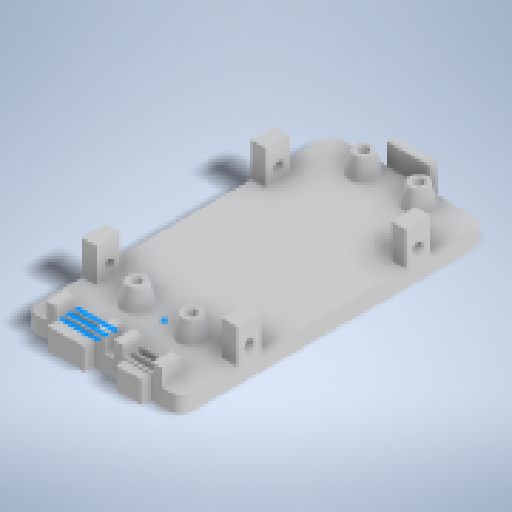
# Autodesk Inventor part: Base
Saved by Autodesk Inventor 2023 (Build 270158000, 158)
## iProperties
Created: 2022-06-08
Part Number: Base
Material: Generic
Document SubType Name: Modeling
Designer: siwat
Density: 1 g/cm^3
Appearance: Default
Author: siwat
Autodesk Inventor part; units mm, degrees
(part 1 of 3)
ref_plane "YZ Plane" through (0, 0, 0) normal (1, 0, 0) x (0, 1, 0)
ref_plane "XZ Plane" through (0, 0, 0) normal (0, 1, 0) x (-1, 0, 0)
ref_plane "XY Plane" through (0, 0, 0) normal (0, 0, 1) x (1, 0, 0)
sketch "Sketch1" plane through (0, 0, 0) normal (0, 1, 0) x (-1, 0, 0)
  line L0 (12.1706, 0.6153) -> (-9.8294, 0.6153)
  line L1 (-9.8294, 0.6153) -> (-9.8294, -51.3847)
  line L2 (-9.8294, -51.3847) -> (12.1706, -51.3847)
  line L3 (12.1706, -51.3847) -> (12.1706, 0.6153)
  line L4 (1.9706, -2.0847) -> (1.9706, 0.1153) projected
  arc A0 (1.7706, -2.2847) -> (1.9706, -2.0847) centre (1.7706, -2.0847) ccw projected
  line L5 (0.5706, -2.2847) -> (1.7706, -2.2847) projected
  arc A1 (0.3706, -2.0847) -> (0.5706, -2.2847) centre (0.5706, -2.0847) ccw projected
  line L6 (0.3706, 0.1153) -> (0.3706, -2.0847) projected
  line L7 (0.3706, 0.1153) -> (-0.5694, 0.1153) projected
  line L8 (-0.5694, -1.4847) -> (-0.5694, 0.1153) projected
  arc A2 (-2.1694, -1.4847) -> (-0.5694, -1.4847) centre (-1.3694, -1.4847) ccw projected
  line L9 (-2.1694, 0.1153) -> (-2.1694, -1.4847) projected
  line L10 (-2.1694, 0.1153) -> (-9.3294, 0.1153) projected
  line L11 (-9.3294, 0.1153) -> (-9.3294, -0.4547) projected
  line L12 (-9.3294, -0.4547) -> (-7.7294, -0.4547) projected
  arc A3 (-7.7294, -2.0547) -> (-7.7294, -0.4547) centre (-7.7294, -1.2547) ccw projected
  line L13 (-7.7294, -2.0547) -> (-9.3294, -2.0547) projected
  line L14 (-9.3294, -2.0547) -> (-9.3294, -2.9947) projected
  line L15 (-9.3294, -2.9947) -> (-7.7294, -2.9947) projected
  arc A4 (-7.7294, -4.5947) -> (-7.7294, -2.9947) centre (-7.7294, -3.7947) ccw projected
  line L16 (-7.7294, -4.5947) -> (-9.3294, -4.5947) projected
  line L17 (-9.3294, -4.5947) -> (-9.3294, -5.5347) projected
  line L18 (-9.3294, -5.5347) -> (-7.1294, -5.5347) projected
  arc A5 (-6.9294, -5.7347) -> (-7.1294, -5.5347) centre (-7.1294, -5.7347) ccw projected
  line L19 (-6.9294, -5.7347) -> (-6.9294, -6.9347) projected
  arc A6 (-7.1294, -7.1347) -> (-6.9294, -6.9347) centre (-7.1294, -6.9347) ccw projected
  line L20 (-7.1294, -7.1347) -> (-9.3294, -7.1347) projected
  line L21 (-9.3294, -7.1347) -> (-9.3294, -8.0747) projected
  line L22 (-9.3294, -8.0747) -> (-7.7294, -8.0747) projected
  arc A7 (-7.7294, -9.6747) -> (-7.7294, -8.0747) centre (-7.7294, -8.8747) ccw projected
  line L23 (-7.7294, -9.6747) -> (-9.3294, -9.6747) projected
  line L24 (-9.3294, -9.6747) -> (-9.3294, -10.6147) projected
  line L25 (-9.3294, -10.6147) -> (-7.7294, -10.6147) projected
  arc A8 (-7.7294, -12.2147) -> (-7.7294, -10.6147) centre (-7.7294, -11.4147) ccw projected
  line L26 (-7.7294, -12.2147) -> (-9.3294, -12.2147) projected
  line L27 (-9.3294, -12.2147) -> (-9.3294, -13.1547) projected
  line L28 (-9.3294, -13.1547) -> (-7.7294, -13.1547) projected
  arc A9 (-7.7294, -14.7547) -> (-7.7294, -13.1547) centre (-7.7294, -13.9547) ccw projected
  line L29 (-7.7294, -14.7547) -> (-9.3294, -14.7547) projected
  line L30 (-9.3294, -14.7547) -> (-9.3294, -15.6947) projected
  line L31 (-9.3294, -15.6947) -> (-7.7294, -15.6947) projected
  arc A10 (-7.7294, -17.2947) -> (-7.7294, -15.6947) centre (-7.7294, -16.4947) ccw projected
  line L32 (-7.7294, -17.2947) -> (-9.3294, -17.2947) projected
  line L33 (-9.3294, -17.2947) -> (-9.3294, -18.2347) projected
  line L34 (-9.3294, -18.2347) -> (-7.1294, -18.2347) projected
  arc A11 (-6.9294, -18.4347) -> (-7.1294, -18.2347) centre (-7.1294, -18.4347) ccw projected
  line L35 (-6.9294, -18.4347) -> (-6.9294, -19.6347) projected
  arc A12 (-7.1294, -19.8347) -> (-6.9294, -19.6347) centre (-7.1294, -19.6347) ccw projected
  line L36 (-7.1294, -19.8347) -> (-9.3294, -19.8347) projected
  line L37 (-9.3294, -19.8347) -> (-9.3294, -20.7747) projected
  line L38 (-9.3294, -20.7747) -> (-7.7294, -20.7747) projected
  arc A13 (-7.7294, -22.3747) -> (-7.7294, -20.7747) centre (-7.7294, -21.5747) ccw projected
  line L39 (-7.7294, -22.3747) -> (-9.3294, -22.3747) projected
  line L40 (-9.3294, -22.3747) -> (-9.3294, -23.3147) projected
  line L41 (-9.3294, -23.3147) -> (-7.7294, -23.3147) projected
  arc A14 (-7.7294, -24.9147) -> (-7.7294, -23.3147) centre (-7.7294, -24.1147) ccw projected
  line L42 (-7.7294, -24.9147) -> (-9.3294, -24.9147) projected
  line L43 (-9.3294, -24.9147) -> (-9.3294, -25.8547) projected
  line L44 (-9.3294, -25.8547) -> (-7.7294, -25.8547) projected
  arc A15 (-7.7294, -27.4547) -> (-7.7294, -25.8547) centre (-7.7294, -26.6547) ccw projected
  line L45 (-7.7294, -27.4547) -> (-9.3294, -27.4547) projected
  line L46 (-9.3294, -27.4547) -> (-9.3294, -28.3947) projected
  line L47 (-9.3294, -28.3947) -> (-7.7294, -28.3947) projected
  arc A16 (-7.7294, -29.9947) -> (-7.7294, -28.3947) centre (-7.7294, -29.1947) ccw projected
  line L48 (-7.7294, -29.9947) -> (-9.3294, -29.9947) projected
  line L49 (-9.3294, -29.9947) -> (-9.3294, -30.9347) projected
  line L50 (-9.3294, -30.9347) -> (-7.1294, -30.9347) projected
  arc A17 (-6.9294, -31.1347) -> (-7.1294, -30.9347) centre (-7.1294, -31.1347) ccw projected
  line L51 (-6.9294, -31.1347) -> (-6.9294, -32.3347) projected
  arc A18 (-7.1294, -32.5347) -> (-6.9294, -32.3347) centre (-7.1294, -32.3347) ccw projected
  line L52 (-7.1294, -32.5347) -> (-9.3294, -32.5347) projected
  line L53 (-9.3294, -32.5347) -> (-9.3294, -33.4747) projected
  line L54 (-9.3294, -33.4747) -> (-7.7294, -33.4747) projected
  arc A19 (-7.7294, -35.0747) -> (-7.7294, -33.4747) centre (-7.7294, -34.2747) ccw projected
  line L55 (-7.7294, -35.0747) -> (-9.3294, -35.0747) projected
  line L56 (-9.3294, -35.0747) -> (-9.3294, -36.0147) projected
  line L57 (-9.3294, -36.0147) -> (-7.7294, -36.0147) projected
  arc A20 (-7.7294, -37.6147) -> (-7.7294, -36.0147) centre (-7.7294, -36.8147) ccw projected
  line L58 (-7.7294, -37.6147) -> (-9.3294, -37.6147) projected
  line L59 (-9.3294, -37.6147) -> (-9.3294, -38.5547) projected
  line L60 (-9.3294, -38.5547) -> (-7.7294, -38.5547) projected
  arc A21 (-7.7294, -40.1547) -> (-7.7294, -38.5547) centre (-7.7294, -39.3547) ccw projected
  line L61 (-7.7294, -40.1547) -> (-9.3294, -40.1547) projected
  line L62 (-9.3294, -40.1547) -> (-9.3294, -41.0947) projected
  line L63 (-9.3294, -41.0947) -> (-7.7294, -41.0947) projected
  arc A22 (-7.7294, -42.6947) -> (-7.7294, -41.0947) centre (-7.7294, -41.8947) ccw projected
  line L64 (-7.7294, -42.6947) -> (-9.3294, -42.6947) projected
  line L65 (-9.3294, -42.6947) -> (-9.3294, -43.6347) projected
  line L66 (-9.3294, -43.6347) -> (-7.1294, -43.6347) projected
  arc A23 (-6.9294, -43.8347) -> (-7.1294, -43.6347) centre (-7.1294, -43.8347) ccw projected
  line L67 (-6.9294, -43.8347) -> (-6.9294, -45.0347) projected
  arc A24 (-7.1294, -45.2347) -> (-6.9294, -45.0347) centre (-7.1294, -45.0347) ccw projected
  line L68 (-7.1294, -45.2347) -> (-9.3294, -45.2347) projected
  line L69 (-9.3294, -45.2347) -> (-9.3294, -46.1747) projected
  line L70 (-9.3294, -46.1747) -> (-7.7294, -46.1747) projected
  arc A25 (-7.7294, -47.7747) -> (-7.7294, -46.1747) centre (-7.7294, -46.9747) ccw projected
  line L71 (-7.7294, -47.7747) -> (-9.3294, -47.7747) projected
  line L72 (-9.3294, -47.7747) -> (-9.3294, -48.7147) projected
  line L73 (-9.3294, -48.7147) -> (-7.7294, -48.7147) projected
  arc A26 (-7.7294, -50.3147) -> (-7.7294, -48.7147) centre (-7.7294, -49.5147) ccw projected
  line L74 (-7.7294, -50.3147) -> (-9.3294, -50.3147) projected
  line L75 (-9.3294, -50.3147) -> (-9.3294, -50.8847) projected
  line L76 (-9.3294, -50.8847) -> (11.6706, -50.8847) projected
  line L77 (11.6706, -50.8847) -> (11.6706, -50.3147) projected
  line L78 (10.0706, -50.3147) -> (11.6706, -50.3147) projected
  arc A27 (10.0706, -48.7147) -> (10.0706, -50.3147) centre (10.0706, -49.5147) ccw projected
  line L79 (11.6706, -48.7147) -> (10.0706, -48.7147) projected
  line L80 (11.6706, -48.7147) -> (11.6706, -47.7747) projected
  line L81 (10.0706, -47.7747) -> (11.6706, -47.7747) projected
  arc A28 (10.0706, -46.1747) -> (10.0706, -47.7747) centre (10.0706, -46.9747) ccw projected
  line L82 (11.6706, -46.1747) -> (10.0706, -46.1747) projected
  line L83 (11.6706, -46.1747) -> (11.6706, -45.2347) projected
  line L84 (9.4706, -45.2347) -> (11.6706, -45.2347) projected
  arc A29 (9.2706, -45.0347) -> (9.4706, -45.2347) centre (9.4706, -45.0347) ccw projected
  line L85 (9.2706, -43.8347) -> (9.2706, -45.0347) projected
  arc A30 (9.4706, -43.6347) -> (9.2706, -43.8347) centre (9.4706, -43.8347) ccw projected
  line L86 (11.6706, -43.6347) -> (9.4706, -43.6347) projected
  line L87 (11.6706, -43.6347) -> (11.6706, -42.6947) projected
  line L88 (10.0706, -42.6947) -> (11.6706, -42.6947) projected
  arc A31 (10.0706, -41.0947) -> (10.0706, -42.6947) centre (10.0706, -41.8947) ccw projected
  line L89 (11.6706, -41.0947) -> (10.0706, -41.0947) projected
  line L90 (11.6706, -41.0947) -> (11.6706, -40.1547) projected
  line L91 (10.0706, -40.1547) -> (11.6706, -40.1547) projected
  arc A32 (10.0706, -38.5547) -> (10.0706, -40.1547) centre (10.0706, -39.3547) ccw projected
  line L92 (11.6706, -38.5547) -> (10.0706, -38.5547) projected
  line L93 (11.6706, -38.5547) -> (11.6706, -37.6147) projected
  line L94 (10.0706, -37.6147) -> (11.6706, -37.6147) projected
  arc A33 (10.0706, -36.0147) -> (10.0706, -37.6147) centre (10.0706, -36.8147) ccw projected
  line L95 (11.6706, -36.0147) -> (10.0706, -36.0147) projected
  line L96 (11.6706, -36.0147) -> (11.6706, -35.0747) projected
  line L97 (10.0706, -35.0747) -> (11.6706, -35.0747) projected
  arc A34 (10.0706, -33.4747) -> (10.0706, -35.0747) centre (10.0706, -34.2747) ccw projected
  line L98 (11.6706, -33.4747) -> (10.0706, -33.4747) projected
  line L99 (11.6706, -33.4747) -> (11.6706, -32.5347) projected
  line L100 (9.4706, -32.5347) -> (11.6706, -32.5347) projected
  arc A35 (9.2706, -32.3347) -> (9.4706, -32.5347) centre (9.4706, -32.3347) ccw projected
  line L101 (9.2706, -31.1347) -> (9.2706, -32.3347) projected
  arc A36 (9.4706, -30.9347) -> (9.2706, -31.1347) centre (9.4706, -31.1347) ccw projected
  line L102 (11.6706, -30.9347) -> (9.4706, -30.9347) projected
  line L103 (11.6706, -30.9347) -> (11.6706, -29.9947) projected
  line L104 (10.0706, -29.9947) -> (11.6706, -29.9947) projected
  arc A37 (10.0706, -28.3947) -> (10.0706, -29.9947) centre (10.0706, -29.1947) ccw projected
  line L105 (11.6706, -28.3947) -> (10.0706, -28.3947) projected
  line L106 (11.6706, -28.3947) -> (11.6706, -27.4547) projected
  line L107 (10.0706, -27.4547) -> (11.6706, -27.4547) projected
  arc A38 (10.0706, -25.8547) -> (10.0706, -27.4547) centre (10.0706, -26.6547) ccw projected
  line L108 (11.6706, -25.8547) -> (10.0706, -25.8547) projected
  line L109 (11.6706, -25.8547) -> (11.6706, -24.9147) projected
  line L110 (10.0706, -24.9147) -> (11.6706, -24.9147) projected
  arc A39 (10.0706, -23.3147) -> (10.0706, -24.9147) centre (10.0706, -24.1147) ccw projected
  line L111 (11.6706, -23.3147) -> (10.0706, -23.3147) projected
  line L112 (11.6706, -23.3147) -> (11.6706, -22.3747) projected
  line L113 (10.0706, -22.3747) -> (11.6706, -22.3747) projected
  arc A40 (10.0706, -20.7747) -> (10.0706, -22.3747) centre (10.0706, -21.5747) ccw projected
  line L114 (11.6706, -20.7747) -> (10.0706, -20.7747) projected
  line L115 (11.6706, -20.7747) -> (11.6706, -19.8347) projected
  line L116 (9.4706, -19.8347) -> (11.6706, -19.8347) projected
  arc A41 (9.2706, -19.6347) -> (9.4706, -19.8347) centre (9.4706, -19.6347) ccw projected
  line L117 (9.2706, -18.4347) -> (9.2706, -19.6347) projected
  arc A42 (9.4706, -18.2347) -> (9.2706, -18.4347) centre (9.4706, -18.4347) ccw projected
  line L118 (11.6706, -18.2347) -> (9.4706, -18.2347) projected
  line L119 (11.6706, -18.2347) -> (11.6706, -17.2947) projected
  line L120 (10.0706, -17.2947) -> (11.6706, -17.2947) projected
  arc A43 (10.0706, -15.6947) -> (10.0706, -17.2947) centre (10.0706, -16.4947) ccw projected
  line L121 (11.6706, -15.6947) -> (10.0706, -15.6947) projected
  line L122 (11.6706, -15.6947) -> (11.6706, -14.7547) projected
  line L123 (10.0706, -14.7547) -> (11.6706, -14.7547) projected
  arc A44 (10.0706, -13.1547) -> (10.0706, -14.7547) centre (10.0706, -13.9547) ccw projected
  line L124 (11.6706, -13.1547) -> (10.0706, -13.1547) projected
  line L125 (11.6706, -13.1547) -> (11.6706, -12.2147) projected
  line L126 (10.0706, -12.2147) -> (11.6706, -12.2147) projected
  arc A45 (10.0706, -10.6147) -> (10.0706, -12.2147) centre (10.0706, -11.4147) ccw projected
  line L127 (11.6706, -10.6147) -> (10.0706, -10.6147) projected
  line L128 (11.6706, -10.6147) -> (11.6706, -9.6747) projected
  line L129 (10.0706, -9.6747) -> (11.6706, -9.6747) projected
  arc A46 (10.0706, -8.0747) -> (10.0706, -9.6747) centre (10.0706, -8.8747) ccw projected
  line L130 (11.6706, -8.0747) -> (10.0706, -8.0747) projected
  line L131 (11.6706, -8.0747) -> (11.6706, -7.1347) projected
  line L132 (9.4706, -7.1347) -> (11.6706, -7.1347) projected
  arc A47 (9.2706, -6.9347) -> (9.4706, -7.1347) centre (9.4706, -6.9347) ccw projected
  line L133 (9.2706, -5.7347) -> (9.2706, -6.9347) projected
  arc A48 (9.4706, -5.5347) -> (9.2706, -5.7347) centre (9.4706, -5.7347) ccw projected
  line L134 (11.6706, -5.5347) -> (9.4706, -5.5347) projected
  line L135 (11.6706, -5.5347) -> (11.6706, -4.5947) projected
  line L136 (10.0706, -4.5947) -> (11.6706, -4.5947) projected
  arc A49 (10.0706, -2.9947) -> (10.0706, -4.5947) centre (10.0706, -3.7947) ccw projected
  line L137 (11.6706, -2.9947) -> (10.0706, -2.9947) projected
  line L138 (11.6706, -2.9947) -> (11.6706, -2.0547) projected
  line L139 (10.0706, -2.0547) -> (11.6706, -2.0547) projected
  arc A50 (10.0706, -0.4547) -> (10.0706, -2.0547) centre (10.0706, -1.2547) ccw projected
  line L140 (11.6706, -0.4547) -> (10.0706, -0.4547) projected
  line L141 (11.6706, -0.4547) -> (11.6706, 0.1153) projected
  line L142 (11.6706, 0.1153) -> (4.5106, 0.1153) projected
  line L143 (4.5106, -1.4847) -> (4.5106, 0.1153) projected
  arc A51 (2.9106, -1.4847) -> (4.5106, -1.4847) centre (3.7106, -1.4847) ccw projected
  line L144 (2.9106, 0.1153) -> (2.9106, -1.4847) projected
  line L145 (2.9106, 0.1153) -> (1.9706, 0.1153) projected
  circle A52 centre (-4.5294, -48.8847) radius 1.9 projected
  circle A53 centre (6.8706, -48.8847) radius 1.9 projected
  circle A54 centre (-4.5294, -1.8847) radius 1.9 projected
  circle A55 centre (6.8706, -1.8847) radius 1.9 projected
  line L146 (15.1706, -52.3847) -> (-12.8294, -52.3847)
  line L147 (-14.8294, -50.3847) -> (-14.8294, 8.6153)
  line L148 (-12.8294, 10.6153) -> (15.1706, 10.6153)
  line L149 (17.1706, 8.6153) -> (17.1706, -50.3847)
  arc A56 (17.1706, 8.6153) -> (15.1706, 10.6153) centre (15.1706, 8.6153) ccw
  arc A57 (-12.8294, 10.6153) -> (-14.8294, 8.6153) centre (-12.8294, 8.6153) ccw
  arc A58 (-14.8294, -50.3847) -> (-12.8294, -52.3847) centre (-12.8294, -50.3847) ccw
  arc A59 (15.1706, -52.3847) -> (17.1706, -50.3847) centre (15.1706, -50.3847) ccw
  circle A60 centre (-4.5294, -1.8847) radius 0.75
  circle A61 centre (6.8706, -1.8847) radius 0.75
  circle A62 centre (-4.5294, -48.8847) radius 0.75
  circle A63 centre (6.8706, -48.8847) radius 0.75
  point P0 (11.6706, -2.5247)
  point P1 (-9.3294, -48.2447)
  point P2 (17.1706, -52.3847)
  point P3 (-14.8294, 10.6153)
  point P4 (-14.8294, -52.3847)
  point P5 (17.1706, 10.6153)
  dimension "d0" = 0.5
  dimension "d1" = 0.5
  dimension "d2" = 0.5
  dimension "d3" = 0.5
  dimension "d4" = 1
  dimension "d5" = 5
  dimension "d6" = 5
  dimension "d7" = 10
  dimension "d10" = 2
  dimension "d11" = 1.5
  dimension "d12" = 1.5
  dimension "d13" = 1.5
  dimension "d14" = 1.5
  constraints: 16 end point, 8 centre point, 8 point on circle, 8 point on line, 8 tangent, 4 coincident, 4 parallel, 3 equal radius, 2 horizontal, 2 midpoint, 2 perpendicular
  measures "d0" distance from line of L3 point (11.671, -2.525)
  measures "d1" distance between parallel lines of L0 L142
  measures "d2" distance between parallel lines of L2 L76
  measures "d3" distance from line of point (-9.329, -48.245) L1
  measures "d4" distance between parallel lines of L146 L2
  measures "d5" distance between parallel lines of L3 L149
  measures "d6" distance between parallel lines of L147 L1
  measures "d7" distance between parallel lines of L148 L0
  measures "d10" radius of A56
  measures "d11" diameter of A60
  measures "d12" diameter of A61
  measures "d13" diameter of A62
  measures "d14" diameter of A63
extrude "Extrusion1" add sketch "Sketch1" against normal blind 3.5 contours L3 L2 L1 L0 | L4 L145 L144 A51 L143 L142 L141 L140 A50 L139 L138 L137 A49 L136 L135 L134 A48 L133 A47 L132 L131 L130 A46 L129 L128 L127 A45 L126 L125 L124 A44 L123 L122 L121 A43 L120 L119 L118 A42 L117 A41 L116 L115 L114 A40 L113 L112 L111 A39 L110 L109 L108 A38 L107 L106 L105 A37 L104 L103 L102 A36 L101 A35 L100 L99 L98 A34 L97 L96 L95 A33 L94 L93 L92 A32 L91 L90 L89 A31 L88 L87 L86 A30 L85 A29 L84 L83 L82 A28 L81 L80 L79 A27 L78 L77 L76 L75 L74 A26 L73 L72 L71 A25 L70 L69 L68 A24 L67 A23 L66 L65 L64 A22 L63 L62 L61 A21 L60 L59 L58 A20 L57 L56 L55 A19 L54 L53 L52 A18 L51 A17 L50 L49 L48 A16 L47 L46 L45 A15 L44 L43 L42 A14 L41 L40 L39 A13 L38 L37 L36 A12 L35 A11 L34 L33 L32 A10 L31 L30 L29 A9 L28 L27 L26 A8 L25 L24 L23 A7 L22 L21 L20 A6 L19 A5 L18 L17 L16 A4 L15 L14 L13 A3 L12 L11 L10 L9 A2 L8 L7 L6 A1 L5 A0 | A52 | A53 | A54 | A55 | L146 A58 L147 A57 L148 A56 L149 A59 | A60 | A61 | A62 | A63
sketch "Sketch2" plane through (0, 0, 0) normal (0, 1, 0) x (1, 0, 0)
  line L0 (-1.9706, 2.0847) -> (-1.9706, -0.1153) projected
  arc A0 (-1.7706, 2.2847) -> (-1.9706, 2.0847) centre (-1.7706, 2.0847) ccw projected
  line L1 (-0.5706, 2.2847) -> (-1.7706, 2.2847) projected
  arc A1 (-0.3706, 2.0847) -> (-0.5706, 2.2847) centre (-0.5706, 2.0847) ccw projected
  line L2 (-0.3706, -0.1153) -> (-0.3706, 2.0847) projected
  line L3 (-0.3706, -0.1153) -> (0.5694, -0.1153) projected
  line L4 (0.5694, 1.4847) -> (0.5694, -0.1153) projected
  arc A2 (2.1694, 1.4847) -> (0.5694, 1.4847) centre (1.3694, 1.4847) ccw projected
  line L5 (2.1694, -0.1153) -> (2.1694, 1.4847) projected
  line L6 (2.1694, -0.1153) -> (9.3294, -0.1153) projected
  line L7 (9.3294, -0.1153) -> (9.3294, 0.4547) projected
  line L8 (9.3294, 0.4547) -> (7.7294, 0.4547) projected
  arc A3 (7.7294, 2.0547) -> (7.7294, 0.4547) centre (7.7294, 1.2547) ccw projected
  line L9 (7.7294, 2.0547) -> (9.3294, 2.0547) projected
  line L10 (9.3294, 2.0547) -> (9.3294, 2.9947) projected
  line L11 (9.3294, 2.9947) -> (7.7294, 2.9947) projected
  arc A4 (7.7294, 4.5947) -> (7.7294, 2.9947) centre (7.7294, 3.7947) ccw projected
  line L12 (7.7294, 4.5947) -> (9.3294, 4.5947) projected
  line L13 (9.3294, 4.5947) -> (9.3294, 5.5347) projected
  line L14 (9.3294, 5.5347) -> (7.1294, 5.5347) projected
  arc A5 (6.9294, 5.7347) -> (7.1294, 5.5347) centre (7.1294, 5.7347) ccw projected
  line L15 (6.9294, 5.7347) -> (6.9294, 6.9347) projected
  arc A6 (7.1294, 7.1347) -> (6.9294, 6.9347) centre (7.1294, 6.9347) ccw projected
  line L16 (7.1294, 7.1347) -> (9.3294, 7.1347) projected
  line L17 (9.3294, 7.1347) -> (9.3294, 8.0747) projected
  line L18 (9.3294, 8.0747) -> (7.7294, 8.0747) projected
  arc A7 (7.7294, 9.6747) -> (7.7294, 8.0747) centre (7.7294, 8.8747) ccw projected
  line L19 (7.7294, 9.6747) -> (9.3294, 9.6747) projected
  line L20 (9.3294, 9.6747) -> (9.3294, 10.6147) projected
  line L21 (9.3294, 10.6147) -> (7.7294, 10.6147) projected
  arc A8 (7.7294, 12.2147) -> (7.7294, 10.6147) centre (7.7294, 11.4147) ccw projected
  line L22 (7.7294, 12.2147) -> (9.3294, 12.2147) projected
  line L23 (9.3294, 12.2147) -> (9.3294, 13.1547) projected
  line L24 (9.3294, 13.1547) -> (7.7294, 13.1547) projected
  arc A9 (7.7294, 14.7547) -> (7.7294, 13.1547) centre (7.7294, 13.9547) ccw projected
  line L25 (7.7294, 14.7547) -> (9.3294, 14.7547) projected
  line L26 (9.3294, 14.7547) -> (9.3294, 15.6947) projected
  line L27 (9.3294, 15.6947) -> (7.7294, 15.6947) projected
  arc A10 (7.7294, 17.2947) -> (7.7294, 15.6947) centre (7.7294, 16.4947) ccw projected
  line L28 (7.7294, 17.2947) -> (9.3294, 17.2947) projected
  line L29 (9.3294, 17.2947) -> (9.3294, 18.2347) projected
  line L30 (9.3294, 18.2347) -> (7.1294, 18.2347) projected
  arc A11 (6.9294, 18.4347) -> (7.1294, 18.2347) centre (7.1294, 18.4347) ccw projected
  line L31 (6.9294, 18.4347) -> (6.9294, 19.6347) projected
  arc A12 (7.1294, 19.8347) -> (6.9294, 19.6347) centre (7.1294, 19.6347) ccw projected
  line L32 (7.1294, 19.8347) -> (9.3294, 19.8347) projected
  line L33 (9.3294, 19.8347) -> (9.3294, 20.7747) projected
  line L34 (9.3294, 20.7747) -> (7.7294, 20.7747) projected
  arc A13 (7.7294, 22.3747) -> (7.7294, 20.7747) centre (7.7294, 21.5747) ccw projected
  line L35 (7.7294, 22.3747) -> (9.3294, 22.3747) projected
  line L36 (9.3294, 22.3747) -> (9.3294, 23.3147) projected
  line L37 (9.3294, 23.3147) -> (7.7294, 23.3147) projected
  arc A14 (7.7294, 24.9147) -> (7.7294, 23.3147) centre (7.7294, 24.1147) ccw projected
  line L38 (7.7294, 24.9147) -> (9.3294, 24.9147) projected
  line L39 (9.3294, 24.9147) -> (9.3294, 25.8547) projected
  line L40 (9.3294, 25.8547) -> (7.7294, 25.8547) projected
  arc A15 (7.7294, 27.4547) -> (7.7294, 25.8547) centre (7.7294, 26.6547) ccw projected
  line L41 (7.7294, 27.4547) -> (9.3294, 27.4547) projected
  line L42 (9.3294, 27.4547) -> (9.3294, 28.3947) projected
  line L43 (9.3294, 28.3947) -> (7.7294, 28.3947) projected
  arc A16 (7.7294, 29.9947) -> (7.7294, 28.3947) centre (7.7294, 29.1947) ccw projected
  line L44 (7.7294, 29.9947) -> (9.3294, 29.9947) projected
  line L45 (9.3294, 29.9947) -> (9.3294, 30.9347) projected
  line L46 (9.3294, 30.9347) -> (7.1294, 30.9347) projected
  arc A17 (6.9294, 31.1347) -> (7.1294, 30.9347) centre (7.1294, 31.1347) ccw projected
  line L47 (6.9294, 31.1347) -> (6.9294, 32.3347) projected
  arc A18 (7.1294, 32.5347) -> (6.9294, 32.3347) centre (7.1294, 32.3347) ccw projected
  line L48 (7.1294, 32.5347) -> (9.3294, 32.5347) projected
  line L49 (9.3294, 32.5347) -> (9.3294, 33.4747) projected
  line L50 (9.3294, 33.4747) -> (7.7294, 33.4747) projected
  arc A19 (7.7294, 35.0747) -> (7.7294, 33.4747) centre (7.7294, 34.2747) ccw projected
  line L51 (7.7294, 35.0747) -> (9.3294, 35.0747) projected
  line L52 (9.3294, 35.0747) -> (9.3294, 36.0147) projected
  line L53 (9.3294, 36.0147) -> (7.7294, 36.0147) projected
  arc A20 (7.7294, 37.6147) -> (7.7294, 36.0147) centre (7.7294, 36.8147) ccw projected
  line L54 (7.7294, 37.6147) -> (9.3294, 37.6147) projected
  line L55 (9.3294, 37.6147) -> (9.3294, 38.5547) projected
  line L56 (9.3294, 38.5547) -> (7.7294, 38.5547) projected
  arc A21 (7.7294, 40.1547) -> (7.7294, 38.5547) centre (7.7294, 39.3547) ccw projected
  line L57 (7.7294, 40.1547) -> (9.3294, 40.1547) projected
  line L58 (9.3294, 40.1547) -> (9.3294, 41.0947) projected
  line L59 (9.3294, 41.0947) -> (7.7294, 41.0947) projected
  arc A22 (7.7294, 42.6947) -> (7.7294, 41.0947) centre (7.7294, 41.8947) ccw projected
  line L60 (7.7294, 42.6947) -> (9.3294, 42.6947) projected
  line L61 (9.3294, 42.6947) -> (9.3294, 43.6347) projected
  line L62 (9.3294, 43.6347) -> (7.1294, 43.6347) projected
  arc A23 (6.9294, 43.8347) -> (7.1294, 43.6347) centre (7.1294, 43.8347) ccw projected
  line L63 (6.9294, 43.8347) -> (6.9294, 45.0347) projected
  arc A24 (7.1294, 45.2347) -> (6.9294, 45.0347) centre (7.1294, 45.0347) ccw projected
  line L64 (7.1294, 45.2347) -> (9.3294, 45.2347) projected
  line L65 (9.3294, 45.2347) -> (9.3294, 46.1747) projected
  line L66 (9.3294, 46.1747) -> (7.7294, 46.1747) projected
  arc A25 (7.7294, 47.7747) -> (7.7294, 46.1747) centre (7.7294, 46.9747) ccw projected
  line L67 (7.7294, 47.7747) -> (9.3294, 47.7747) projected
  line L68 (9.3294, 47.7747) -> (9.3294, 48.7147) projected
  line L69 (9.3294, 48.7147) -> (7.7294, 48.7147) projected
  arc A26 (7.7294, 50.3147) -> (7.7294, 48.7147) centre (7.7294, 49.5147) ccw projected
  line L70 (7.7294, 50.3147) -> (9.3294, 50.3147) projected
  line L71 (9.3294, 50.3147) -> (9.3294, 50.8847) projected
  line L72 (9.3294, 50.8847) -> (-11.6706, 50.8847) projected
  line L73 (-11.6706, 50.8847) -> (-11.6706, 50.3147) projected
  line L74 (-10.0706, 50.3147) -> (-11.6706, 50.3147) projected
  arc A27 (-10.0706, 48.7147) -> (-10.0706, 50.3147) centre (-10.0706, 49.5147) ccw projected
  line L75 (-11.6706, 48.7147) -> (-10.0706, 48.7147) projected
  line L76 (-11.6706, 48.7147) -> (-11.6706, 47.7747) projected
  line L77 (-10.0706, 47.7747) -> (-11.6706, 47.7747) projected
  arc A28 (-10.0706, 46.1747) -> (-10.0706, 47.7747) centre (-10.0706, 46.9747) ccw projected
  line L78 (-11.6706, 46.1747) -> (-10.0706, 46.1747) projected
  line L79 (-11.6706, 46.1747) -> (-11.6706, 45.2347) projected
  line L80 (-9.4706, 45.2347) -> (-11.6706, 45.2347) projected
  arc A29 (-9.2706, 45.0347) -> (-9.4706, 45.2347) centre (-9.4706, 45.0347) ccw projected
  line L81 (-9.2706, 43.8347) -> (-9.2706, 45.0347) projected
  arc A30 (-9.4706, 43.6347) -> (-9.2706, 43.8347) centre (-9.4706, 43.8347) ccw projected
  line L82 (-11.6706, 43.6347) -> (-9.4706, 43.6347) projected
  line L83 (-11.6706, 43.6347) -> (-11.6706, 42.6947) projected
  line L84 (-10.0706, 42.6947) -> (-11.6706, 42.6947) projected
  arc A31 (-10.0706, 41.0947) -> (-10.0706, 42.6947) centre (-10.0706, 41.8947) ccw projected
  line L85 (-11.6706, 41.0947) -> (-10.0706, 41.0947) projected
  line L86 (-11.6706, 41.0947) -> (-11.6706, 40.1547) projected
  line L87 (-10.0706, 40.1547) -> (-11.6706, 40.1547) projected
  arc A32 (-10.0706, 38.5547) -> (-10.0706, 40.1547) centre (-10.0706, 39.3547) ccw projected
  line L88 (-11.6706, 38.5547) -> (-10.0706, 38.5547) projected
  line L89 (-11.6706, 38.5547) -> (-11.6706, 37.6147) projected
  line L90 (-10.0706, 37.6147) -> (-11.6706, 37.6147) projected
  arc A33 (-10.0706, 36.0147) -> (-10.0706, 37.6147) centre (-10.0706, 36.8147) ccw projected
  line L91 (-11.6706, 36.0147) -> (-10.0706, 36.0147) projected
  line L92 (-11.6706, 36.0147) -> (-11.6706, 35.0747) projected
  line L93 (-10.0706, 35.0747) -> (-11.6706, 35.0747) projected
  arc A34 (-10.0706, 33.4747) -> (-10.0706, 35.0747) centre (-10.0706, 34.2747) ccw projected
  line L94 (-11.6706, 33.4747) -> (-10.0706, 33.4747) projected
  line L95 (-11.6706, 33.4747) -> (-11.6706, 32.5347) projected
  line L96 (-9.4706, 32.5347) -> (-11.6706, 32.5347) projected
  arc A35 (-9.2706, 32.3347) -> (-9.4706, 32.5347) centre (-9.4706, 32.3347) ccw projected
  line L97 (-9.2706, 31.1347) -> (-9.2706, 32.3347) projected
  arc A36 (-9.4706, 30.9347) -> (-9.2706, 31.1347) centre (-9.4706, 31.1347) ccw projected
  line L98 (-11.6706, 30.9347) -> (-9.4706, 30.9347) projected
  line L99 (-11.6706, 30.9347) -> (-11.6706, 29.9947) projected
  line L100 (-10.0706, 29.9947) -> (-11.6706, 29.9947) projected
  arc A37 (-10.0706, 28.3947) -> (-10.0706, 29.9947) centre (-10.0706, 29.1947) ccw projected
  line L101 (-11.6706, 28.3947) -> (-10.0706, 28.3947) projected
  line L102 (-11.6706, 28.3947) -> (-11.6706, 27.4547) projected
  line L103 (-10.0706, 27.4547) -> (-11.6706, 27.4547) projected
  arc A38 (-10.0706, 25.8547) -> (-10.0706, 27.4547) centre (-10.0706, 26.6547) ccw projected
  line L104 (-11.6706, 25.8547) -> (-10.0706, 25.8547) projected
  line L105 (-11.6706, 25.8547) -> (-11.6706, 24.9147) projected
  line L106 (-10.0706, 24.9147) -> (-11.6706, 24.9147) projected
  arc A39 (-10.0706, 23.3147) -> (-10.0706, 24.9147) centre (-10.0706, 24.1147) ccw projected
  line L107 (-11.6706, 23.3147) -> (-10.0706, 23.3147) projected
  line L108 (-11.6706, 23.3147) -> (-11.6706, 22.3747) projected
  line L109 (-10.0706, 22.3747) -> (-11.6706, 22.3747) projected
  arc A40 (-10.0706, 20.7747) -> (-10.0706, 22.3747) centre (-10.0706, 21.5747) ccw projected
  line L110 (-11.6706, 20.7747) -> (-10.0706, 20.7747) projected
  line L111 (-11.6706, 20.7747) -> (-11.6706, 19.8347) projected
  line L112 (-9.4706, 19.8347) -> (-11.6706, 19.8347) projected
  arc A41 (-9.2706, 19.6347) -> (-9.4706, 19.8347) centre (-9.4706, 19.6347) ccw projected
  line L113 (-9.2706, 18.4347) -> (-9.2706, 19.6347) projected
  arc A42 (-9.4706, 18.2347) -> (-9.2706, 18.4347) centre (-9.4706, 18.4347) ccw projected
  line L114 (-11.6706, 18.2347) -> (-9.4706, 18.2347) projected
  line L115 (-11.6706, 18.2347) -> (-11.6706, 17.2947) projected
  line L116 (-10.0706, 17.2947) -> (-11.6706, 17.2947) projected
  arc A43 (-10.0706, 15.6947) -> (-10.0706, 17.2947) centre (-10.0706, 16.4947) ccw projected
  line L117 (-11.6706, 15.6947) -> (-10.0706, 15.6947) projected
  line L118 (-11.6706, 15.6947) -> (-11.6706, 14.7547) projected
  line L119 (-10.0706, 14.7547) -> (-11.6706, 14.7547) projected
  arc A44 (-10.0706, 13.1547) -> (-10.0706, 14.7547) centre (-10.0706, 13.9547) ccw projected
  line L120 (-11.6706, 13.1547) -> (-10.0706, 13.1547) projected
  line L121 (-11.6706, 13.1547) -> (-11.6706, 12.2147) projected
  line L122 (-10.0706, 12.2147) -> (-11.6706, 12.2147) projected
  arc A45 (-10.0706, 10.6147) -> (-10.0706, 12.2147) centre (-10.0706, 11.4147) ccw projected
  line L123 (-11.6706, 10.6147) -> (-10.0706, 10.6147) projected
  line L124 (-11.6706, 10.6147) -> (-11.6706, 9.6747) projected
  line L125 (-10.0706, 9.6747) -> (-11.6706, 9.6747) projected
  arc A46 (-10.0706, 8.0747) -> (-10.0706, 9.6747) centre (-10.0706, 8.8747) ccw projected
  line L126 (-11.6706, 8.0747) -> (-10.0706, 8.0747) projected
  line L127 (-11.6706, 8.0747) -> (-11.6706, 7.1347) projected
  line L128 (-9.4706, 7.1347) -> (-11.6706, 7.1347) projected
  arc A47 (-9.2706, 6.9347) -> (-9.4706, 7.1347) centre (-9.4706, 6.9347) ccw projected
  line L129 (-9.2706, 5.7347) -> (-9.2706, 6.9347) projected
  arc A48 (-9.4706, 5.5347) -> (-9.2706, 5.7347) centre (-9.4706, 5.7347) ccw projected
  line L130 (-11.6706, 5.5347) -> (-9.4706, 5.5347) projected
  line L131 (-11.6706, 5.5347) -> (-11.6706, 4.5947) projected
  line L132 (-10.0706, 4.5947) -> (-11.6706, 4.5947) projected
  arc A49 (-10.0706, 2.9947) -> (-10.0706, 4.5947) centre (-10.0706, 3.7947) ccw projected
  line L133 (-11.6706, 2.9947) -> (-10.0706, 2.9947) projected
  line L134 (-11.6706, 2.9947) -> (-11.6706, 2.0547) projected
  line L135 (-10.0706, 2.0547) -> (-11.6706, 2.0547) projected
  arc A50 (-10.0706, 0.4547) -> (-10.0706, 2.0547) centre (-10.0706, 1.2547) ccw projected
  line L136 (-11.6706, 0.4547) -> (-10.0706, 0.4547) projected
  line L137 (-11.6706, 0.4547) -> (-11.6706, -0.1153) projected
  line L138 (-11.6706, -0.1153) -> (-4.5106, -0.1153) projected
  line L139 (-4.5106, 1.4847) -> (-4.5106, -0.1153) projected
  arc A51 (-2.9106, 1.4847) -> (-4.5106, 1.4847) centre (-3.7106, 1.4847) ccw projected
  line L140 (-2.9106, -0.1153) -> (-2.9106, 1.4847) projected
  line L141 (-2.9106, -0.1153) -> (-1.9706, -0.1153) projected
  circle A52 centre (4.5294, 48.8847) radius 1.9 projected
  circle A53 centre (-6.8706, 48.8847) radius 1.9 projected
  circle A54 centre (4.5294, 1.8847) radius 1.9 projected
  circle A55 centre (-6.8706, 1.8847) radius 1.9 projected
  circle A56 centre (4.5294, 1.8847) radius 1.9
  circle A57 centre (-6.8706, 1.8847) radius 2
  circle A58 centre (-6.8706, 48.8847) radius 1.9
  circle A59 centre (4.5294, 48.8847) radius 1.9
  circle A60 centre (4.5294, 48.8847) radius 1
  circle A61 centre (-6.8706, 48.8847) radius 1
  circle A62 centre (4.5294, 1.8847) radius 1
  circle A63 centre (-6.8706, 1.8847) radius 1
  point P0 (0, 0)
  dimension "d15" = 2
  dimension "d16" = 2
  dimension "d17" = 2
  dimension "d18" = 2
  constraints: 8 centre point, 8 coincident, 3 concentric, 1 tangent
  measures "d15" diameter of A60
  measures "d16" diameter of A61
  measures "d17" diameter of A62
  measures "d18" diameter of A63
extrude "Extrusion2" add sketch "Sketch2" along normal blind 4 contours A52 | A53 | A54 | A55
chamfer "Chamfer1" distance 1 distance2 4 4 edges at (2.6294, 0, -48.8847) (-8.7706, 0, -48.8847) (-8.7706, 0, -1.8847) (2.6294, 0, -1.8847) measured on face at (2.1294, 0, -1.8847) measured on face at (-9.2706, 0, -1.8847) measured on face at (2.1294, 0, -48.8847) measured on face at (-9.2706, 0, -48.8847)
sketch "Sketch3" plane through (0, 0, 0) normal (0, 1, 0) x (1, 0, 0)
  line L0 (14.8294, 50.3847) -> (14.8294, -8.6153) projected
  line L1 (14.8294, 40.8847) -> (11.8294, 40.8847)
  line L2 (11.8294, 40.8847) -> (11.8294, 35.8847)
  line L3 (11.8294, 35.8847) -> (14.8294, 35.8847)
  line L4 (14.8294, 35.8847) -> (14.8294, 40.8847)
  line L5 (14.8294, 5.8847) -> (11.8294, 5.8847)
  line L6 (11.8294, 5.8847) -> (11.8294, 0.8847)
  line L7 (11.8294, 0.8847) -> (14.8294, 0.8847)
  line L8 (14.8294, 0.8847) -> (14.8294, 5.8847)
  line L9 (-17.1706, 50.3847) -> (-17.1706, -8.6153) projected
  line L10 (-17.1706, 40.8847) -> (-14.1706, 40.8847)
  line L11 (-14.1706, 40.8847) -> (-14.1706, 35.8847)
  line L12 (-14.1706, 35.8847) -> (-17.1706, 35.8847)
  line L13 (-17.1706, 35.8847) -> (-17.1706, 40.8847)
  line L14 (-17.1706, 5.8847) -> (-14.1706, 5.8847)
  line L15 (-14.1706, 5.8847) -> (-14.1706, 0.8847)
  line L16 (-14.1706, 0.8847) -> (-17.1706, 0.8847)
  line L17 (-17.1706, 0.8847) -> (-17.1706, 5.8847)
  line L18 (-15.1706, -10.6153) -> (12.8294, -10.6153) projected
  line L19 (12.8294, 52.3847) -> (-15.1706, 52.3847) projected
  point P0 (0, 0)
  point P1 (13.3294, 5.8847)
  point P2 (13.3294, 35.8847)
  point P3 (13.3294, 40.8847)
  dimension "d27" = 3
  dimension "d28" = 5
  dimension "d29" = 3
  dimension "d30" = 5
  dimension "d31" = 3
  dimension "d32" = 5
  dimension "d33" = 3
  dimension "d34" = 5
  dimension "d35" = 30
  dimension "d36" = 63
  dimension "d37" = 11.5
  constraints: 32 end point, 8 parallel, 4 horizontal, 4 perpendicular, 4 point on line, 3 midpoint, 2 collinear
  measures "d27" distance of L3.end L2.end
  measures "d28" distance of L2.end L1.end
  measures "d29" distance of L7.end L6.end
  measures "d30" distance of L6.end L5.end
  measures "d31" distance of L11.end L12.end
  measures "d32" distance of L10.end L11.end
  measures "d33" distance of L15.end L16.end
  measures "d34" distance of L14.end L15.end
  measures "d35" distance of point (13.329, 5.885) point (13.329, 35.885)
  measures "d36" distance between parallel lines of L18 L19
  measures "d37" distance from line of L19 point (13.329, 40.885)
extrude "Extrusion3" add sketch "Sketch3" along normal blind 5
sketch "Sketch4" plane through (-17.1706, -3.5, -50.3847) normal (-1, 0, 0) x (0, 0, 1)
  circle A0 centre (11.9956, 6) radius 1
  line L0 (14.5, 3.5) -> (14.5, 8.5) projected
  line L1 (9.5, 8.5) -> (14.5, 8.5) projected
  line L2 (9.9901, 8.5) -> (9.5, 8.5)
  line L3 (9.5, 8.5) -> (9.5, 5.2905)
  line L4 (9.5, 3.5) -> (9.5, 8.5) projected
  line L5 (14.0011, 8.5) -> (14.5, 8.5)
  circle A1 centre (47, 6) radius 1
  line L6 (44.5, 8.5) -> (49.5, 8.5) projected
  point P0 (50.3847, 3.5)
  dimension "d40" = 2
  dimension "d41" = 2.5
  dimension "d42" = 2
  dimension "d43" = 2.5
  constraints: 6 end point, 3 point on line, 2 centre point, 1 collinear, 1 perpendicular
  measures "d40" diameter of A0
  measures "d41" distance from line of L1 A0.centre
  measures "d42" diameter of A1
  measures "d43" distance from line of L6 A1.centre
extrude "Extrusion4" cut sketch "Sketch4" against normal up to surface (3 mm away)
sketch "Sketch5" plane through (14.8294, -3.5, 8.6153) normal (1, 0, 0) x (0, 0, -1)
  circle A0 centre (47.0044, 6) radius 1 projected
  circle A1 centre (12, 6) radius 1 projected
  point P0 (8.6153, 3.5)
extrude "Extrusion5" cut sketch "Sketch5" against normal up to surface (3 mm away)
sketch "Sketch6" plane through (0, 0, 0) normal (0, 1, 0) x (1, 0, 0)
  line L0 (-15.1706, -10.6153) -> (12.8294, -10.6153) projected
  line L1 (-11.1706, -10.6153) -> (-3.1706, -10.6153)
  line L2 (-3.1706, -10.6153) -> (-3.1706, -6.6153)
  line L3 (-3.1706, -6.6153) -> (-11.1706, -6.6153)
  line L4 (-11.1706, -6.6153) -> (-11.1706, -10.6153)
  line L5 (2.8294, -10.6153) -> (8.8294, -10.6153)
  line L6 (8.8294, -10.6153) -> (8.8294, -6.6153)
  line L7 (8.8294, -6.6153) -> (2.8294, -6.6153)
  line L8 (2.8294, -6.6153) -> (2.8294, -10.6153)
  line L9 (-11.1706, -6.6153) -> (-13.1706, -6.6153)
  line L10 (-13.1706, -6.6153) -> (-13.1706, -10.6153)
  line L11 (-13.1706, -10.6153) -> (-11.1706, -10.6153)
  line L12 (-11.1706, -10.6153) -> (-11.1706, -6.6153)
  line L13 (-3.1706, -6.6153) -> (-1.1706, -6.6153)
  line L14 (-1.1706, -6.6153) -> (-1.1706, -10.6153)
  line L15 (-1.1706, -10.6153) -> (-3.1706, -10.6153)
  line L16 (-3.1706, -10.6153) -> (-3.1706, -6.6153)
  line L17 (2.8294, -6.6153) -> (0.8294, -6.6153)
  line L18 (0.8294, -6.6153) -> (0.8294, -10.6153)
  line L19 (0.8294, -10.6153) -> (2.8294, -10.6153)
  line L20 (2.8294, -10.6153) -> (2.8294, -6.6153)
  line L21 (8.8294, -6.6153) -> (10.8294, -6.6153)
  line L22 (10.8294, -6.6153) -> (10.8294, -10.6153)
  line L23 (10.8294, -10.6153) -> (8.8294, -10.6153)
  line L24 (8.8294, -10.6153) -> (8.8294, -6.6153)
  line L25 (14.8294, -8.6153) -> (14.8294, 0.8847) projected
  line L26 (-17.1706, -8.6153) -> (-17.1706, 50.3847) projected
  line L27 (12.8294, -10.6153) -> (-15.1706, -10.6153) projected
  line L28 (-11.4706, -10.6153) -> (-11.4706, -6.6153)
  line L29 (2.5294, -6.6153) -> (2.5294, -10.6153)
  line L30 (-2.8706, -10.6153) -> (-2.8706, -6.6153)
  line L31 (9.1294, -6.6153) -> (9.1294, -10.6153)
  point P0 (0, 0)
  point P1 (-3.1706, -10.6153)
  dimension "d48" = 8
  dimension "d49" = 4
  dimension "d50" = 6
  dimension "d51" = 4
  dimension "d52" = 2
  dimension "d53" = 2
  dimension "d54" = 2
  dimension "d55" = 2
  dimension "d56" = 4
  dimension "d57" = 4
  dimension "d80" = 0.3
  dimension "d81" = 0.3
  dimension "d82" = 0.3
  dimension "d83" = 0.3
  constraints: 56 end point, 12 parallel, 11 point on line, 10 perpendicular, 6 horizontal, 1 midpoint, 3 other
  measures "d48" distance of L3.end L2.end
  measures "d49" distance of L2.end L1.end
  measures "d50" distance of L7.end L6.end
  measures "d51" distance of L6.end L5.end
  measures "d52" distance of L11.end L10.end
  measures "d53" distance of L14.end L15.end
  measures "d54" distance of L19.end L18.end
  measures "d55" distance of L22.end L23.end
  measures "d56" distance between parallel lines of L22 L25
  measures "d57" distance between parallel lines of L26 L10
  measures "d80" distance between parallel lines of L4 L28
  measures "d81" distance between parallel lines of L2 L30
  measures "d82" distance between parallel lines of L8 L29
  measures "d83" distance between parallel lines of L6 L31
extrude "Extrusion6" add sketch "Sketch6" along normal blind 3.5 contours L10 L9 L28 L0 | L28 L9 L4 L0 | L2 L13 L30 L0 | L30 L13 L14 L0 | L18 L17 L29 L0 | L29 L17 L8 L0 | L6 L21 L31 L0 | L31 L21 L22 L0
sketch "Sketch7" plane through (0, 0, 0) normal (0, 1, 0) x (1, 0, 0)
  line L0 (-13.1706, -6.6153) -> (-11.1706, -6.6153) projected
  line L1 (10.8294, -6.6153) -> (8.8294, -6.6153) projected
  line L2 (-11.1706, -6.6153) -> (8.8294, -6.6153)
  line L3 (-3.1706, -10.6153) -> (-3.1706, -6.6153) projected
  line L4 (-11.1706, -6.6153) -> (-3.1706, -6.6153)
  line L5 (-3.1706, -6.6153) -> (-3.1706, -7.1153)
  line L6 (-3.1706, -7.1153) -> (-11.1706, -7.1153)
  line L7 (-11.1706, -7.1153) -> (-11.1706, -6.6153)
  line L8 (8.8294, -6.6153) -> (8.8294, -10.6153) projected
  line L9 (2.8294, -6.6153) -> (8.8294, -6.6153)
  line L10 (8.8294, -6.6153) -> (8.8294, -7.1153)
  line L11 (8.8294, -7.1153) -> (2.8294, -7.1153)
  line L12 (2.8294, -7.1153) -> (2.8294, -6.6153)
  line L13 (12.8294, -10.6153) -> (-15.1706, -10.6153) projected
  line L14 (-11.1706, -10.6153) -> (-3.1706, -10.6153)
  line L15 (-3.1706, -10.6153) -> (-3.1706, -10.1153)
  line L16 (-3.1706, -10.1153) -> (-11.1706, -10.1153)
  line L17 (-11.1706, -10.1153) -> (-11.1706, -10.6153)
  line L18 (2.8294, -10.6153) -> (8.8294, -10.6153)
  line L19 (8.8294, -10.6153) -> (8.8294, -10.1153)
  line L20 (8.8294, -10.1153) -> (2.8294, -10.1153)
  line L21 (2.8294, -10.1153) -> (2.8294, -10.6153)
  line L22 (-11.1706, -6.6153) -> (-11.1706, -10.6153) projected
  line L23 (-11.1706, -8.6153) -> (8.8294, -8.6153)
  line L24 (-11.1706, -8.6153) -> (-3.1706, -8.6153)
  line L25 (-3.1706, -8.6153) -> (-3.1706, -8.3653)
  line L26 (-3.1706, -8.3653) -> (-11.1706, -8.3653)
  line L27 (-11.1706, -8.3653) -> (-11.1706, -8.6153)
  line L28 (-11.1706, -8.6153) -> (-3.1706, -8.6153)
  line L29 (-3.1706, -8.6153) -> (-3.1706, -8.8653)
  line L30 (-3.1706, -8.8653) -> (-11.1706, -8.8653)
  line L31 (-11.1706, -8.8653) -> (-11.1706, -8.6153)
  line L32 (2.8294, -6.6153) -> (2.8294, -10.6153) projected
  line L33 (2.8294, -8.6153) -> (8.8294, -8.6153)
  line L34 (8.8294, -8.6153) -> (8.8294, -8.3653)
  line L35 (8.8294, -8.3653) -> (2.8294, -8.3653)
  line L36 (2.8294, -8.3653) -> (2.8294, -8.6153)
  line L37 (8.8294, -8.6153) -> (2.8294, -8.6153)
  line L38 (2.8294, -8.6153) -> (2.8294, -8.8653)
  line L39 (2.8294, -8.8653) -> (8.8294, -8.8653)
  line L40 (8.8294, -8.8653) -> (8.8294, -8.6153)
  point P0 (0, 0)
  point P1 (2.8294, -10.6153)
  point P2 (2.8294, -8.3653)
  point P3 (8.8294, -8.8653)
  dimension "d60" = 0.5
  dimension "d61" = 0.5
  dimension "d62" = 0.25
  dimension "d63" = 0.25
  dimension "d64" = 0.25
  dimension "d65" = 0.25
  constraints: 68 end point, 16 parallel, 11 point on line, 8 horizontal, 8 perpendicular, 3 midpoint, 1 collinear
  measures "d60" distance of L4.end L5.end
  measures "d61" distance between parallel lines of L13 L16
  measures "d62" distance of L25.end L24.end
  measures "d63" distance of L28.end L29.end
  measures "d64" distance of L34.end L33.end
  measures "d65" distance of L38.end L37.end
extrude "Extrusion7" add sketch "Sketch7" along normal blind 1.5 contours L2 L3 L6 L7 | L2 L8 L11 L12 | L26 L3 L23 L22 | L23 L3 L30 L22 | L35 L8 L23 L32 | L23 L8 L39 L32 | L16 L3 L13 L17 | L20 L8 L13 L21
sketch "Sketch8" plane through (12.8294, 0, -52.3847) normal (0, 0, -1) x (-1, 0, 0)
  line L0 (28, -3.5) -> (18.6537, -3.5) projected
  line L1 (28, -3.5) -> (28, 9.6375) projected
  line L2 (0, 9.6375) -> (28, 9.6375) projected
  line L3 (0, -3.5) -> (0, 9.6375) projected
  line L4 (18.6537, -3.5) -> (9.5348, -3.5)
  line L5 (9.5348, 4.3788) -> (18.6537, 4.3788)
  line L6 (18.4537, 4.3788) -> (18.4537, -3.5)
  line L7 (9.7348, 4.3788) -> (9.7348, -3.5)
  line L8 (28, -3.5) -> (0, -3.5) projected
  line L9 (19.6069, 7.2201) -> (18.9116, 8.0955) projected
  line L10 (18.9116, 8.0955) -> (18.5765, 8.0955) projected
  line L11 (18.5765, 8.0955) -> (18.5765, 7.2201) projected
  line L12 (18.5765, 7.2201) -> (18.2841, 7.2201) projected
  line L13 (18.2841, 7.2201) -> (18.2841, 9.4201) projected
  line L14 (18.2841, 9.4201) -> (18.851, 9.4201) projected
  spline S0 degree 2 poles (18.851, 9.4201) (19.04, 9.4201) (19.295, 9.3791) (19.4108, 9.3043) knots 0 0 0 1 2 2 2 projected
  spline S1 degree 2 poles (19.4108, 9.3043) (19.5267, 9.2294) (19.6604, 8.9958) (19.6604, 8.8229) knots 0 0 0 1 2 2 2 projected
  spline S2 degree 2 poles (19.6604, 8.8229) (19.6604, 8.5822) (19.4144, 8.256) (19.204, 8.1775) knots 0 0 0 1 2 2 2 projected
  line L15 (19.204, 8.1775) -> (19.9867, 7.2201) projected
  line L16 (19.9867, 7.2201) -> (19.6069, 7.2201) projected
  line L17 (15.3335, 9.1599) -> (14.5954, 9.1599) projected
  line L18 (14.5954, 9.1599) -> (14.5954, 9.4201) projected
  line L19 (14.5954, 9.4201) -> (16.364, 9.4201) projected
  line L20 (16.364, 9.4201) -> (16.364, 9.1599) projected
  line L21 (16.364, 9.1599) -> (15.6259, 9.1599) projected
  line L22 (15.6259, 9.1599) -> (15.6259, 7.2201) projected
  line L23 (15.6259, 7.2201) -> (15.3335, 7.2201) projected
  line L24 (15.3335, 7.2201) -> (15.3335, 9.1599) projected
  line L25 (10.5823, 7.2201) -> (10.5823, 9.1153) projected
  line L26 (10.5823, 9.1153) -> (10.0082, 7.8263) projected
  line L27 (10.0082, 7.8263) -> (9.83, 7.8263) projected
  line L28 (9.83, 7.8263) -> (9.2612, 9.1153) projected
  line L29 (9.2612, 9.1153) -> (9.2612, 7.2201) projected
  line L30 (9.2612, 7.2201) -> (8.9885, 7.2201) projected
  line L31 (8.9885, 7.2201) -> (8.9885, 9.4201) projected
  line L32 (8.9885, 9.4201) -> (9.3878, 9.4201) projected
  line L33 (9.3878, 9.4201) -> (9.9369, 8.1953) projected
  line L34 (9.9369, 8.1953) -> (10.4682, 9.4201) projected
  line L35 (10.4682, 9.4201) -> (10.8747, 9.4201) projected
  line L36 (10.8747, 9.4201) -> (10.8747, 7.2201) projected
  line L37 (10.8747, 7.2201) -> (10.5823, 7.2201) projected
  line L38 (11.8249, 9.4201) -> (12.1851, 9.4201) projected
  line L39 (12.1851, 9.4201) -> (12.9267, 7.2201) projected
  line L40 (12.9267, 7.2201) -> (12.6183, 7.2201) projected
  line L41 (12.6183, 7.2201) -> (12.4186, 7.8352) projected
  line L42 (12.4186, 7.8352) -> (11.5789, 7.8352) projected
  line L43 (11.5789, 7.8352) -> (11.3792, 7.2201) projected
  line L44 (11.3792, 7.2201) -> (11.0833, 7.2201) projected
  line L45 (11.0833, 7.2201) -> (11.8249, 9.4201) projected
  line L46 (13.0266, 7.3521) -> (13.0266, 7.7193) projected
  line L47 (13.0266, 7.7193) -> (13.048, 7.7193) projected
  spline S3 degree 2 poles (13.048, 7.7193) (13.1924, 7.5838) (13.5578, 7.4341) (13.7272, 7.4341) knots 0 0 0 1 2 2 2 projected
  spline S4 degree 2 poles (13.7272, 7.4341) (13.9697, 7.4341) (14.2175, 7.6355) (14.2175, 7.8013) knots 0 0 0 1 2 2 2 projected
  spline S5 degree 2 poles (14.2175, 7.8013) (14.2175, 7.9333) (14.0873, 8.0973) (13.9465, 8.1383) knots 0 0 0 1 2 2 2 projected
  spline S6 degree 2 poles (13.9465, 8.1383) (13.8449, 8.1668) (13.6755, 8.206) (13.5489, 8.2381) knots 0 0 0 1 2 2 2 projected
  spline S7 degree 2 poles (13.5489, 8.2381) (13.4348, 8.2684) (13.2548, 8.3594) (13.1852, 8.4325) knots 0 0 0 1 2 2 2 projected
  spline S8 degree 2 poles (13.1852, 8.4325) (13.1175, 8.5056) (13.0426, 8.7017) (13.0426, 8.83) knots 0 0 0 1 2 2 2 projected
  spline S9 degree 2 poles (13.0426, 8.83) (13.0426, 9.0975) (13.4598, 9.4594) (13.7825, 9.4594) knots 0 0 0 1 2 2 2 projected
  spline S10 degree 2 poles (13.7825, 9.4594) (13.9679, 9.4594) (14.2959, 9.3863) (14.4368, 9.3167) knots 0 0 0 1 2 2 2 projected
  line L48 (14.4368, 9.3167) -> (14.4368, 8.9673) projected
  line L49 (14.4368, 8.9673) -> (14.4154, 8.9673) projected
  spline S11 degree 2 poles (14.4154, 8.9673) (14.3102, 9.0636) (13.9822, 9.2062) (13.8021, 9.2062) knots 0 0 0 1 2 2 2 projected
  spline S12 degree 2 poles (13.8021, 9.2062) (13.5988, 9.2062) (13.3475, 9.0154) (13.3475, 8.8603) knots 0 0 0 1 2 2 2 projected
  spline S13 degree 2 poles (13.3475, 8.8603) (13.3475, 8.7213) (13.4954, 8.5555) (13.6345, 8.518) knots 0 0 0 1 2 2 2 projected
  spline S14 degree 2 poles (13.6345, 8.518) (13.7272, 8.4931) (13.9964, 8.4289) (14.0856, 8.4022) knots 0 0 0 1 2 2 2 projected
  spline S15 degree 2 poles (14.0856, 8.4022) (14.312, 8.3326) (14.5223, 8.0527) (14.5223, 7.8477) knots 0 0 0 1 2 2 2 projected
  spline S16 degree 2 poles (14.5223, 7.8477) (14.5223, 7.7176) (14.4172, 7.468) (14.3227, 7.3806) knots 0 0 0 1 2 2 2 projected
  spline S17 degree 2 poles (14.3227, 7.3806) (14.2175, 7.2843) (13.9501, 7.1809) (13.7486, 7.1809) knots 0 0 0 1 2 2 2 projected
  spline S18 degree 2 poles (13.7486, 7.1809) (13.5097, 7.1809) (13.1745, 7.2808) (13.0266, 7.3521) knots 0 0 0 1 2 2 2 projected
  line L50 (16.5869, 9.4201) -> (17.9632, 9.4201) projected
  line L51 (17.9632, 9.4201) -> (17.9632, 9.1599) projected
  line L52 (17.9632, 9.1599) -> (16.8792, 9.1599) projected
  line L53 (16.8792, 9.1599) -> (16.8792, 8.5573) projected
  line L54 (16.8792, 8.5573) -> (17.8901, 8.5573) projected
  line L55 (17.8901, 8.5573) -> (17.8901, 8.297) projected
  line L56 (17.8901, 8.297) -> (16.8792, 8.297) projected
  line L57 (16.8792, 8.297) -> (16.8792, 7.4804) projected
  line L58 (16.8792, 7.4804) -> (17.9632, 7.4804) projected
  line L59 (17.9632, 7.4804) -> (17.9632, 7.2201) projected
  line L60 (17.9632, 7.2201) -> (16.5869, 7.2201) projected
  line L61 (16.5869, 7.2201) -> (16.5869, 9.4201) projected
  line L62 (18.6537, 6.9181) -> (18.6537, -3.5) projected
  line L63 (9.5348, -3.5) -> (0, -3.5) projected
  line L64 (9.5348, -3.5) -> (9.5348, 6.9181) projected
  line L65 (9.5348, 6.9181) -> (18.6537, 6.9181) projected
  point P0 (12.8294, 0)
  point P1 (9.7348, -3.5)
  constraints: 8 end point, 4 point on line, 1 parallel, 1 perpendicular
ref_plane "Work Plane1" through (-15.1706, -2, -54.1847) normal (0, 0, -1) x (0, 1, 0)
extrude "Extrusion8" add sketch "Sketch8" along normal up to surface (1.8 mm away) contours L4 L7 L5 L6
sketch "Sketch10" plane through (0, -3.5, 0) normal (0, -1, 0) x (1, 0, 0)
  line L0 (12.8294, 10.6153) -> (-15.1706, 10.6153) projected
  line L1 (-10.9467, 10.6153) -> (-3.4875, 10.6153)
  line L2 (-3.4875, 10.6153) -> (-3.4875, 12.4164)
  line L3 (-3.4875, 12.4164) -> (-10.9467, 12.4164)
  line L4 (-10.9467, 12.4164) -> (-10.9467, 10.6153)
  line L5 (3.1637, 10.6153) -> (8.4217, 10.6153)
  line L6 (8.4217, 10.6153) -> (8.4217, 12.4164)
  line L7 (8.4217, 12.4164) -> (3.1637, 12.4164)
  line L8 (3.1637, 12.4164) -> (3.1637, 10.6153)
  point P0 (0, 0)
  point P1 (3.1637, 10.6153)
  point P2 (8.4217, 10.6153)
  point P3 (-3.4875, 10.6153)
  constraints: 16 end point, 4 parallel, 3 point on line, 2 horizontal, 2 perpendicular
extrude "Extrusion9" add sketch "Sketch10" against normal blind 4.5
sketch "Sketch11" plane through (0, 5, 0) normal (0, 1, 0) x (1, 0, 0)
  line L0 (-14.1706, 5.8847) -> (-17.1706, 5.8847) projected
  line L1 (-17.1706, 5.8847) -> (-17.1706, 0.8847) projected
  line L2 (-17.1706, 0.8847) -> (-14.1706, 0.8847) projected
  line L3 (-14.1706, 0.8847) -> (-14.1706, 5.8847) projected
  line L4 (11.8294, 0.8847) -> (14.8294, 0.8847) projected
  line L5 (14.8294, 0.8847) -> (14.8294, 5.8847) projected
  line L6 (14.8294, 5.8847) -> (11.8294, 5.8847) projected
  line L7 (11.8294, 5.8847) -> (11.8294, 0.8847) projected
  line L8 (14.8294, 39.3891) -> (11.8294, 39.3891) projected
  line L9 (14.8294, 40.8847) -> (11.8294, 40.8847) projected
  line L10 (11.8294, 35.8847) -> (14.8294, 35.8847) projected
  line L11 (14.8294, 35.8847) -> (14.8294, 40.8847) projected
  line L12 (14.8294, 40.8847) -> (11.8294, 40.8847) projected
  line L13 (11.8294, 40.8847) -> (11.8294, 35.8847) projected
  line L14 (-14.1706, 40.8847) -> (-17.1706, 40.8847) projected
  line L15 (-17.1706, 40.8847) -> (-17.1706, 35.8847) projected
  line L16 (-17.1706, 35.8847) -> (-14.1706, 35.8847) projected
  line L17 (-14.1706, 35.8847) -> (-14.1706, 40.8847) projected
  point P0 (0, 0)
ref_plane "Work Plane2" through (-17.4706, 8.6375, -52.6847) normal (0, -1, 0) x (1, 0, 0)
extrude "Extrusion10" add sketch "Sketch11" along normal blind 2.1
sketch "Sketch12" plane through (0, 0, 0) normal (0, 1, 0) x (1, 0, 0)
  circle A0 centre (4.5294, 1.8847) radius 1 projected
  circle A1 centre (-6.8706, 1.8847) radius 1 projected
  circle A2 centre (-6.8706, 48.8847) radius 1 projected
  circle A3 centre (4.5294, 48.8847) radius 1 projected
  point P0 (0, 0)
extrude "Extrusion11" cut sketch "Sketch12" against normal blind 3.2
sketch "Sketch13" plane through (0, 1.5, 0) normal (0, 1, 0) x (1, 0, 0)
  line L0 (-11.1706, -8.3653) -> (-3.1706, -8.3653) projected
  line L1 (-11.1706, -7.1153) -> (-3.1706, -7.1153) projected
  line L2 (-3.1706, -6.6153) -> (-3.1706, -7.1153) projected
  line L3 (-3.1706, -6.6153) -> (-11.1706, -6.6153) projected
  line L4 (-11.1706, -7.1153) -> (-11.1706, -6.6153) projected
  line L5 (-11.1706, -8.8653) -> (-11.1706, -8.3653) projected
  line L6 (-11.1706, -8.8653) -> (-3.1706, -8.8653) projected
  line L7 (-3.1706, -8.3653) -> (-3.1706, -8.8653) projected
  line L8 (-3.1706, -8.3653) -> (-11.1706, -8.3653) projected
  line L9 (-11.1706, -10.6153) -> (-3.1706, -10.6153) projected
  line L10 (-3.1706, -10.1153) -> (-3.1706, -10.6153) projected
  line L11 (-3.1706, -10.1153) -> (-11.1706, -10.1153) projected
  line L12 (-11.1706, -10.6153) -> (-11.1706, -10.1153) projected
  point P0 (0, 0)
extrude "Extrusion12" cut sketch "Sketch13" against normal blind 0.475